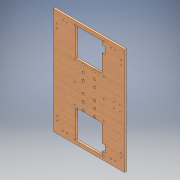
# Autodesk Inventor part: base_robot
Saved by Autodesk Inventor 2017 (Build 210142000, 142)
## iProperties
Created: 2017-04-14
Part Number: base_robot
Material: Generic
Document SubType Name: Modeling
Designer: franc
Density: 1 g/cm^3
Appearance: Default
Author: franc
Autodesk Inventor part; units mm, degrees
ref_plane "YZ Plane" through (0, 0, 0) normal (1, 0, 0) x (0, 1, 0)
ref_plane "XZ Plane" through (0, 0, 0) normal (0, 1, 0) x (-1, 0, 0)
ref_plane "XY Plane" through (0, 0, 0) normal (0, 0, 1) x (1, 0, 0)
sketch "Sketch1" plane through (0, 0, 0) normal (0, 1, 0) x (-1, 0, 0)
  line L0 (21.656, 146.8254) -> (-178.344, 146.8254)
  line L1 (-178.344, 146.8254) -> (-178.344, -153.1746)
  line L2 (-178.344, -153.1746) -> (21.656, -153.1746)
  line L3 (21.656, -153.1746) -> (21.656, 146.8254)
  line L4 (-41.344, 136.8254) -> (-115.344, 136.8254)
  line L5 (-115.344, 56.8254) -> (-41.344, 56.8254)
  line L6 (-41.344, 56.8254) -> (-41.344, 136.8254)
  line L7 (-41.344, -63.1746) -> (-115.344, -63.1746)
  line L8 (-115.344, -143.1746) -> (-41.344, -143.1746)
  line L9 (-41.344, -143.1746) -> (-41.344, -63.1746)
  circle A0 centre (-119.344, 136.8254) radius 1.5
  circle A1 centre (-37.344, 136.8254) radius 1.5
  circle A2 centre (-37.344, -143.1746) radius 1.5
  circle A3 centre (-119.344, -143.1746) radius 1.5
  circle A4 centre (-119.344, 51.8254) radius 1.5
  circle A5 centre (-119.344, -3.1746) radius 1.5
  circle A6 centre (-119.344, -58.1746) radius 1.5
  circle A7 centre (-37.344, 51.8254) radius 1.5
  circle A8 centre (-37.344, -3.1746) radius 1.5
  circle A9 centre (-37.344, -58.1746) radius 1.5
  line L10 (-115.344, 136.8254) -> (-115.344, 126.8254)
  line L11 (-115.344, 126.8254) -> (-123.344, 126.8254)
  line L12 (-123.344, 126.8254) -> (-123.344, 106.8254)
  line L13 (-123.344, 106.8254) -> (-115.344, 106.8254)
  line L14 (-115.344, 106.8254) -> (-115.344, 56.8254)
  line L15 (-115.344, -63.1746) -> (-115.344, -113.1746)
  line L16 (-115.344, -113.1746) -> (-123.344, -113.1746)
  line L17 (-123.344, -113.1746) -> (-123.344, -133.1746)
  line L18 (-123.344, -133.1746) -> (-115.344, -133.1746)
  line L19 (-115.344, -133.1746) -> (-115.344, -143.1746)
  circle A10 centre (-94.344, 52.8254) radius 3
  circle A11 centre (-62.344, 52.8254) radius 3
  circle A12 centre (-62.344, -59.1746) radius 3
  circle A13 centre (-94.344, -59.1746) radius 3
  circle A14 centre (-94.344, 32.8254) radius 3
  circle A15 centre (-94.344, 12.8254) radius 3
  circle A16 centre (-62.344, 32.8254) radius 3
  circle A17 centre (-62.344, 12.8254) radius 3
  circle A18 centre (-94.344, -39.1746) radius 3
  circle A19 centre (-94.344, -19.1746) radius 3
  circle A20 centre (-62.344, -39.1746) radius 3
  circle A21 centre (-62.344, -19.1746) radius 3
  circle A22 centre (-4.844, -138.1746) radius 1.5
  circle A23 centre (-16.844, -138.1746) radius 1.5
  circle A24 centre (11.656, -121.6746) radius 1.5
  circle A25 centre (11.656, -109.6746) radius 1.5
  circle A26 centre (-4.844, 131.8254) radius 1.5
  circle A27 centre (-16.844, 131.8254) radius 1.5
  circle A28 centre (11.656, 115.3254) radius 1.5
  circle A29 centre (11.656, 103.3254) radius 1.5
  circle A30 centre (-139.844, -138.1746) radius 1.5
  circle A31 centre (-151.844, -138.1746) radius 1.5
  circle A32 centre (-168.344, -121.6746) radius 1.5
  circle A33 centre (-168.344, -109.6746) radius 1.5
  circle A34 centre (-139.844, 131.8254) radius 1.5
  circle A35 centre (-151.844, 131.8254) radius 1.5
  circle A36 centre (-168.344, 115.3254) radius 1.5
  circle A37 centre (-168.344, 103.3254) radius 1.5
  circle A38 centre (-164.844, 4.8254) radius 1
  circle A39 centre (-164.844, -11.1746) radius 1
  circle A40 centre (-148.844, -11.1746) radius 1
  circle A41 centre (-148.844, 4.8254) radius 1
  point P0 (0, 0)
  dimension "d0" = 300
  dimension "d1" = 200
  dimension "d2" = 10
  dimension "d3" = 10
  dimension "d4" = 80
  dimension "d5" = 80
  dimension "d6" = 74
  dimension "d7" = 74
  dimension "d10" = 10
  dimension "d12" = 3
  dimension "d13" = 10
  dimension "d15" = 3
  dimension "d16" = 10
  dimension "d18" = 3
  dimension "d19" = 10
  dimension "d21" = 3
  dimension "d22" = 85
  dimension "d23" = 55
  dimension "d24" = 55
  dimension "d25" = 85
  dimension "d28" = 3
  dimension "d29" = 3
  dimension "d30" = 3
  dimension "d31" = 85
  dimension "d32" = 55
  dimension "d33" = 55
  dimension "d34" = 85
  dimension "d37" = 3
  dimension "d38" = 3
  dimension "d39" = 3
  dimension "d42" = 10
  dimension "d43" = 8
  dimension "d45" = 20
  dimension "d46" = 10
  dimension "d47" = 20
  dimension "d48" = 8
  dimension "d49" = 94
  dimension "d50" = 94
  dimension "d51" = 94
  dimension "d52" = 94
  dimension "d55" = 6
  dimension "d56" = 6
  dimension "d59" = 6
  dimension "d60" = 6
  dimension "d63" = 20
  dimension "d64" = 20
  dimension "d65" = 6
  dimension "d66" = 6
  dimension "d71" = 20
  dimension "d72" = 20
  dimension "d75" = 20
  dimension "d76" = 20
  dimension "d77" = 6
  dimension "d78" = 6
  dimension "d81" = 20
  dimension "d82" = 20
  dimension "d83" = 6
  dimension "d84" = 6
  dimension "d91" = 3
  dimension "d92" = 3
  dimension "d93" = 15
  dimension "d94" = 15
  dimension "d95" = 26.5
  dimension "d96" = 12
  constraints: 42 centre point, 40 end point, 9 perpendicular, 5 equal length, 3 horizontal, 2 point on line, 2 vertical
  measures "d0" distance of L2.end L0.start
  measures "d1" distance of L0.start L0.end
  measures "d2" distance between parallel lines of L0 L4
  measures "d3" distance between parallel lines of L2 L8
  measures "d4" distance of L5.end L4.start
  measures "d5" distance of L8.end L7.start
  measures "d6" distance of L5.start L5.end
  measures "d7" distance of L7.start L7.end
  measures "d10" distance from line of A0.centre L0
  measures "d12" diameter of A0
  measures "d13" distance from line of L0 A1.centre
  measures "d15" diameter of A1
  measures "d16" distance from line of L2 A2.centre
  measures "d18" diameter of A2
  measures "d19" distance from line of L2 A3.centre
  measures "d21" diameter of A3
  measures "d22" distance of A7.centre A1.centre
  measures "d23" distance of A8.centre A7.centre
  measures "d24" distance of A9.centre A8.centre
  measures "d25" distance of A2.centre A9.centre
  measures "d28" diameter of A7
  measures "d29" diameter of A8
  measures "d30" diameter of A9
  measures "d31" distance of A4.centre A0.centre
  measures "d32" distance of A5.centre A4.centre
  measures "d33" distance of A6.centre A5.centre
  measures "d34" distance of A3.centre A6.centre
  measures "d37" diameter of A4
  measures "d38" diameter of A5
  measures "d39" diameter of A6
  measures "d42" distance of L4.end L10.end
  measures "d43" distance of L10.end L11.end
  measures "d45" distance of L11.end L12.end
  measures "d46" distance of L18.end L8.start
  measures "d47" distance of L16.end L17.end
  measures "d48" distance of L17.end L18.end
  measures "d49" distance from line of L0 A10.centre
  measures "d50" distance from line of L0 A11.centre
  measures "d51" distance from line of L2 A12.centre
  measures "d52" distance from line of L2 A13.centre
  measures "d55" diameter of A11
  measures "d56" diameter of A10
  measures "d59" diameter of A12
  measures "d60" diameter of A13
  measures "d63" distance of A16.centre A11.centre
  measures "d64" distance of A17.centre A16.centre
  measures "d65" diameter of A16
  measures "d66" diameter of A17
  measures "d71" distance of A14.centre A15.centre
  measures "d72" distance of A10.centre A14.centre
  measures "d75" distance of A19.centre A18.centre
  measures "d76" distance of A13.centre A18.centre
  measures "d77" diameter of A18
  measures "d78" diameter of A19
  measures "d81" distance of A20.centre A21.centre
  measures "d82" distance of A12.centre A20.centre
  measures "d83" diameter of A20
  measures "d84" diameter of A21
  measures "d91" diameter of A22
  measures "d92" diameter of A23
  measures "d93" distance from line of L2 A22.centre
  measures "d94" distance from line of L2 A23.centre
  measures "d95" distance from line of L3 A22.centre
  measures "d96" distance of A23.centre A22.centre
extrude "Extrusion2" add sketch "Sketch1" along normal blind 5
body "Solid2"
